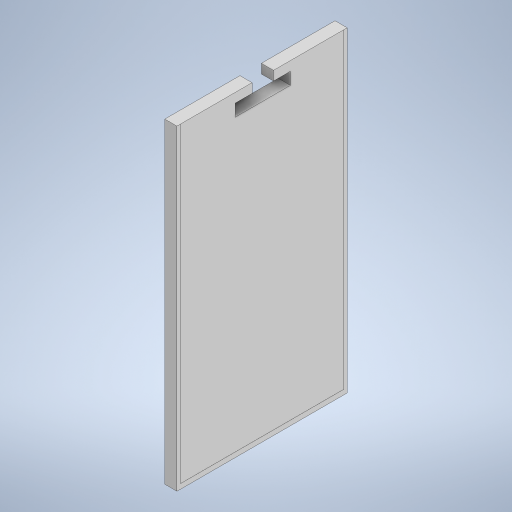
# Autodesk Inventor part: baseplateinverseproto 1
Saved by Autodesk Inventor 2023 (Build 270158000, 158)
## iProperties
Created: 2025-08-30
Part Number: baseplateinverseproto 1
Material: Generic
Document SubType Name: Modeling
Designer: ptato_qo49uko
Density: 1 g/cm^3
Appearance: Default
Author: ptato_qo49uko
Autodesk Inventor part; units mm, degrees
ref_plane "YZ Plane" through (0, 0, 0) normal (1, 0, 0) x (0, 1, 0)
ref_plane "XZ Plane" through (0, 0, 0) normal (0, 1, 0) x (-1, 0, 0)
ref_plane "XY Plane" through (0, 0, 0) normal (0, 0, 1) x (1, 0, 0)
sketch "Sketch1" plane through (0, 0, 0) normal (1, 0, 0) x (0, 1, 0)
  line L0 (82.3549, 41.969) -> (-47.6451, 41.969)
  line L1 (-47.6451, 41.969) -> (-47.6451, -28.031)
  line L2 (-47.6451, -28.031) -> (82.3549, -28.031)
  line L3 (82.3549, -28.031) -> (82.3549, 41.969)
  point P0 (0, 0)
  dimension "d0" = 130
  dimension "d1" = 70
  constraints: 8 end point, 2 parallel, 1 horizontal, 1 perpendicular
  measures "d0" distance of L2.end L1.end
  measures "d1" distance of L1.end L0.end
extrude "Extrusion1" add sketch "Sketch1" along normal blind 5
sketch "Sketch13" plane through (5, 0, 0) normal (1, 0, 0) x (0, 0, -1)
  line L0 (-41.969, -47.6451) -> (28.031, -47.6451) projected
  line L1 (28.031, 82.3549) -> (-41.969, 82.3549) projected
  line L2 (28.031, -47.6451) -> (26.531, -47.6451)
  line L3 (26.531, -47.6451) -> (26.531, 82.3549)
  line L4 (26.531, 82.3549) -> (28.031, 82.3549)
  line L5 (28.031, 82.3549) -> (28.031, -47.6451)
  line L6 (-41.969, 82.3549) -> (-41.969, -47.6451) projected
  line L7 (28.031, 82.3549) -> (-41.969, 82.3549) projected
  line L8 (-41.969, -47.6451) -> (-40.469, -47.6451)
  line L9 (-40.469, -47.6451) -> (-40.469, 82.3549)
  line L10 (-40.469, 82.3549) -> (-41.969, 82.3549)
  line L11 (-41.969, 82.3549) -> (-41.969, -47.6451)
  line L12 (28.031, -47.6451) -> (-41.969, -47.6451)
  line L13 (-41.969, -47.6451) -> (-41.969, -45.6451)
  line L14 (-41.969, -45.6451) -> (28.031, -45.6451)
  line L15 (28.031, -45.6451) -> (28.031, -47.6451)
  point P0 (0, 0)
  point P1 (10.031, 62.3549)
  point P2 (-5.969, 62.3549)
  point P3 (26.531, -45.6451)
  point P4 (-40.469, -45.6451)
  point P5 (18.031, 62.3549)
  dimension "d42" = 1.5
  dimension "d43" = 1.5
  dimension "d44" = 2
  constraints: 24 end point, 6 parallel, 3 horizontal, 3 perpendicular, 1 point on line, 4 other
  measures "d42" distance of L3.end L4.end
  measures "d43" distance of L10.end L9.end
  measures "d44" distance of L12.end L13.end
extrude "Extrusion7" add sketch "Sketch13" along normal blind 0.01 contours L6 L14 L9 L0 | L9 L14 L3 L0 | L6 L1 L9 L14 | L3 L14 L5 L0 | L3 L1 L5 L14
sketch "Sketch18" plane through (5, 0, 0) normal (1, 0, 0) x (0, 0, -1)
  line L0 (-10.769, 82.3549) -> (-2.569, 82.3549)
  line L1 (-2.569, 82.3549) -> (-2.2688, 82.3549)
  line L2 (-10.769, 82.3549) -> (-11.069, 82.3549)
  line L3 (-11.069, 82.3549) -> (-11.069, 78.5449)
  line L4 (-2.2688, 82.3549) -> (-2.2688, 78.5449)
  line L5 (-2.2688, 78.5449) -> (4.6812, 78.5449)
  line L6 (-11.069, 78.5449) -> (-18.019, 78.5449)
  line L7 (-18.019, 78.5449) -> (-18.019, 73.5449)
  line L8 (4.6812, 78.5449) -> (4.6812, 73.5449)
  line L9 (-18.019, 73.5449) -> (-7.137, 73.5449)
  line L10 (-7.137, 73.5449) -> (4.6812, 73.5449)
  line L11 (-2.2688, 82.3549) -> (-11.069, 82.3549)
  line L12 (26.531, 82.3549) -> (26.531, -45.6451) projected
  point P0 (0, 0)
  point P1 (4.531, 82.3549)
  point P2 (-3.669, 82.3549)
  point P3 (11.531, 82.3549)
  dimension "d78" = 7.4
  dimension "d79" = 3.81
  dimension "d81" = 3.81
  dimension "d83" = 6.95
  dimension "d85" = 6.95
  dimension "d86" = 5
  dimension "d87" = 5
  dimension "d88" = 8.8002
  dimension "d91" = 11.8183
  dimension "d92" = 10.8819
  constraints: 24 end point, 3 horizontal, 3 vertical, 1 perpendicular
  measures "d78" distance of point (-3.669, 82.355) L2.end
  measures "d79" distance of L2.end L3.end
  measures "d81" distance of L1.end L4.end
  measures "d83" distance of L4.end L5.end
  measures "d85" distance of L3.end L6.end
  measures "d86" distance of L6.end L7.end
  measures "d87" distance of L5.end L8.end
  measures "d88" distance of L1.end L2.end
  measures "d91" distance of L9.end L8.end
  measures "d92" distance of L7.end L9.end
extrude "Extrusion10" cut sketch "Sketch18" against normal blind 7.9375
body "Solid1"
